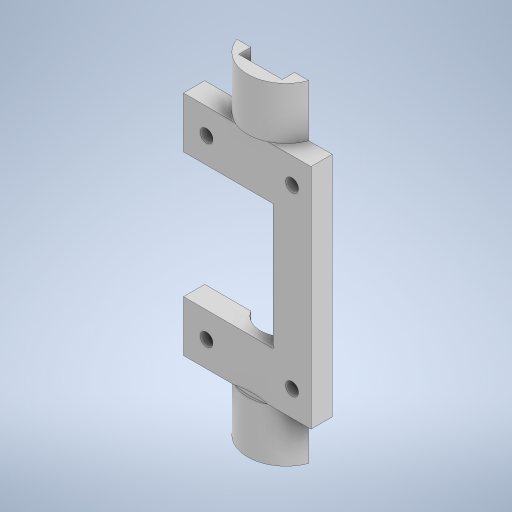
# Autodesk Inventor part: joný=gej
Saved by Autodesk Inventor 2023 (Build 270158000, 158)
## iProperties
Created: 2023-05-01
Part Number: joný=gej
Material: Všeobecné
Document SubType Name: Modeling
Designer: Simak
Density: 1 g/cm^3
Appearance: Výchozí
Author: Simak
Autodesk Inventor part; units mm, degrees
ref_plane "YZ Plane" through (0, 0, 0) normal (1, 0, 0) x (0, 1, 0)
ref_plane "XZ Plane" through (0, 0, 0) normal (0, 1, 0) x (-1, 0, 0)
ref_plane "XY Plane" through (0, 0, 0) normal (0, 0, 1) x (1, 0, 0)
sketch "Náčrt1" plane through (0, 0, 0) normal (0, 0, 1) x (1, 0, 0)
  line L0 (0, 0) -> (0, 26.75)
  line L1 (0, 26.75) -> (-30, 26.75)
  line L2 (-30, 26.75) -> (-30, 14.75)
  line L3 (-30, 14.75) -> (-8.875, 14.75)
  line L4 (-8.875, 14.75) -> (-8.875, 0)
  line L5 (-8.875, 0) -> (0, 0)
  circle A0 centre (-24.5625, 20.75) radius 1.5
  circle A1 centre (-4.4375, 20.75) radius 1.5
  line L6 (-19.125, 26.75) -> (-19.125, 14.75) construction
  dimension "d0" = 30
  dimension "d1" = 26.75
  dimension "d3" = 12
  dimension "d4" = 8.875
  dimension "d5" = 3
  dimension "d6" = 3
  dimension "d7" = 6
  dimension "d9" = 10.875
  dimension "d10" = 5.4375
  dimension "d11" = 4.4375
  constraints: 14 end point, 6 perpendicular, 2 centre point, 2 point on line, 1 horizontal alignment, 1 vertical
  measures "d0" distance of L0.end L1.end
  measures "d1" distance of L0.start L0.end
  measures "d3" distance of L1.end L2.end
  measures "d4" distance between parallel lines of L0 L4
  measures "d5" diameter of A0
  measures "d6" diameter of A1
  measures "d7" distance from line of L1 A0.centre
  measures "d9" distance between parallel lines of L2 L6
  measures "d10" distance from line of L2 A0.centre
  measures "d11" distance from line of L0 A1.centre
extrude "Vysunutí1" add sketch "Náčrt1" along normal blind 5
sketch "Náčrt2" plane through (-30, 26.75, 0) normal (0, 1, 0) x (1, 0, 0)
  circle A0 centre (16, 3.12) radius 6
  line L0 (30, 0) -> (0, 0) projected
  line L1 (21.125, 0) -> (21.125, -5) projected
  line L2 (30, -5) -> (0, -5) projected
  line L3 (10.875, -5) -> (10.875, 0)
  circle A1 centre (16, 3.12) radius 9
  point P0 (24.4419, 0)
  point P1 (7.5581, 0)
  dimension "d1" = 26.75
  dimension "d14" = 12
  dimension "d15" = 10.25
  dimension "d20" = 18
  constraints: 2 centre point, 2 end point, 2 point on circle, 2 point on line, 1 coincident, 1 parallel, 1 vertical
  measures "d14" diameter of A0
  measures "d15" distance between parallel lines of L3 L1
  measures "d20" diameter of A1
extrude "Vysunutí2" add sketch "Náčrt2" along normal blind 3 contours L3 A1 L0 | A0 L1 A1 L2 L3 | L0 A1 L1 | L2 A1
extrude "Vysunutí3" cut sketch "Náčrt2" against normal through all contours L0 A0 picked at (15.3305, -1.5618)
sketch "Náčrt3" plane through (0, 0, 5) normal (0, 0, 1) x (1, 0, 0)
  line L0 (-22.4419, 26.75) -> (-17.8815, 26.75) projected
  line L1 (0, 26.75) -> (-10.1185, 26.75) projected
  arc A0 (-17.8815, 26.75) -> (-10.1185, 26.75) centre (-14, 44.3265) ccw
  line L2 (-10.1185, 26.75) -> (-17.8815, 26.75) projected
  point P0 (0, 0)
  dimension "d21" = 18
  constraints: 2 point on circle, 1 centre point
  measures "d21" radius of A0
revolve "Rotace1" add sketch "Náčrt3" angle 360 about axis through (-10.1185, 26.75, 5) along (-1, 0, 0)
sketch "Náčrt4" plane through (-30, 29.75, 0) normal (0, 1, 0) x (1, 0, 0)
  line L0 (21.125, 0) -> (21.125, -2.88)
  line L1 (21.125, 0) -> (21.125, -5) projected
  arc A0 (10.875, 0) -> (21.125, 0) centre (16, 3.12) ccw projected
  line L2 (10.875, -2.88) -> (10.875, 0)
  line L3 (21.125, -2.88) -> (10.875, -2.88)
  arc A1 (7.5581, 0) -> (24.4419, 0) centre (16, 3.12) ccw projected
  line L4 (24.4419, 0) -> (21.125, 0) projected
  line L5 (10.875, 0) -> (7.5581, 0) projected
  point P0 (30, 0)
  constraints: 6 end point, 1 horizontal, 1 point on line, 1 tangent, 1 vertical
extrude "Vysunutí4" add sketch "Náčrt4" along normal blind 9.25 contours L4 A1 L1 L0 | L1 A1 L5 L2 L3
chamfer "Zkosení1" distance 0.25 angle 45 2 edges at (-16.9394, 29.75, 2.1107) (-11.0606, 29.75, 2.1107)
mirror "Zrcadlit1" about plane through (-8.875, 0, 0) normal (0, -1, 0)
